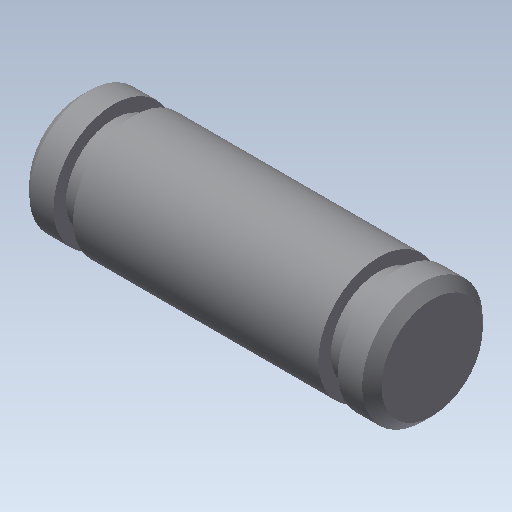
# Autodesk Inventor part: D-12304
Saved by Autodesk Inventor 2020 (Build 240168000, 168)
## iProperties
Created: 2020-01-07
Part Number: D-12304
Material: Generic
Catalog Web Link: www.cadenas.de
Description: Piston Rod Clevis for Original Line Cylinders - Pin-
Vendor: BIMBA
Document SubType Name: Modeling
Designer: psadmin
Manufacturer: BIMBA
Mass: 0.233427 g
Surface Area: 2.57002 cm^2
Volume: 0.233427 cm^3
Density: 1 g/cm^3
Appearance: PSOLRGB-191-191-191
Category: PARTsolutions
Company: BIMBA
PSOL_IDENT_0: {$CADENAS_DATA\23d-libs\bimba\bimba_brand\bimba_imperial\bimba_full_line\original_line_cylinders\acc
PSOL_IDENT_1: essories\piston_rod_clevis_pin.prj},199 {VTYP=3D},{NB=D-12304},{LINA=D-12304},{NN=Piston Rod Clevis
PSOL_IDENT_2: for Original Line Cylinders - Pin},{DATE=23.12.2019 10:36:51},{GEOMDATE=03.04.2013 12:23:00},{VERSIO
PSOL_IDENT_3: N=},{LINEID=20},{WBVAR=},{WBNUMERIC=}  {NB=D-12304},{LINA=D-12304},{KT=DUMMY},{PN=D-12304},{L=0.5460
PSOL_IDENT_4: 0000},{L1=0.38000000},{L2=0.03050000},{L4=0.05250000},{D=0.18700000},{D1=0.14800000},{CH=0.01500000}
PSOL_IDENT_5: ,{R=0.00250000},{COLOR=0.75,0.75,0.75,0.00}
NN: Piston Rod Clevis for Original Line Cylinders - Pin
NB: D-12304
NBSYN: $PN.
LINA: D-12304
PN: D-12304
L: 0.546
L1: 0.38
L2: 0.0305
L4: 0.0525
D: 0.187
D1: 0.148
CH: 0.015
R: 0.0025
SUPPLIER: BIMBA
ARTICLENO: D-12304
BOMINFO: D-12304
CREATOR: CADENAS GmbH
Title: D-12304
Author: Cadenas PARTsolutions
Autodesk Inventor part; units mm, degrees
sketch "Sketch_1" plane through (0, 0, 0) normal (0, 0, 1) x (1, 0, 0)
  line L0 (6.9342, 0) -> (-6.9342, 0)
  line L1 (-6.9342, 0) -> (-6.9342, 1.9939)
  line L2 (-6.9342, 1.9939) -> (-6.5532, 2.3749)
  line L3 (-6.5532, 2.3749) -> (-5.6007, 2.3749)
  line L4 (-5.6007, 2.3749) -> (-5.6007, 1.8796)
  line L5 (-5.6007, 1.8796) -> (-4.826, 1.8796)
  line L6 (-4.826, 1.8796) -> (-4.826, 2.3749)
  line L7 (-4.826, 2.3749) -> (4.826, 2.3749)
  line L8 (4.826, 2.3749) -> (4.826, 1.8796)
  line L9 (4.826, 1.8796) -> (5.6007, 1.8796)
  line L10 (5.6007, 1.8796) -> (5.6007, 2.3749)
  line L11 (5.6007, 2.3749) -> (6.5532, 2.3749)
  line L12 (6.5532, 2.3749) -> (6.9342, 1.9939)
  line L13 (6.9342, 1.9939) -> (6.9342, 0)
  line L14 (6.9342, 0) -> (-6.9342, 0)
  constraints: 30 end point
revolve "Revolution1" add sketch "Sketch_1" angle 360 about axis through (6.9342, 0, 0) along (1, 0, 0)
ref_plane "p1_XY" through (0, 0, 2.3749) normal (1, 0, 0) x (0, 0, -1)
ref_plane "p1_YZ" through (0, 0, 2.3749) normal (0, 0, -1) x (0, 1, 0)
ref_plane "p1_ZX" through (0, 0, 2.3749) normal (0, 1, 0) x (1, 0, 0)
ref_plane "p2_XY" through (0, 0, -2.3749) normal (1, 0, 0) x (0, 0, -1)
ref_plane "p2_YZ" through (0, 0, -2.3749) normal (0, 0, -1) x (0, 1, 0)
ref_plane "p2_ZX" through (0, 0, -2.3749) normal (0, 1, 0) x (1, 0, 0)
ref_plane "pin_XY" through (0, 0, 0) normal (1, 0, 0) x (0, 0, -1)
ref_plane "pin_YZ" through (0, 0, 0) normal (0, 0, -1) x (0, 1, 0)
ref_plane "pin_ZX" through (0, 0, 0) normal (0, 1, 0) x (1, 0, 0)
ref_plane "rr1_XY" through (5.2134, 0, 0) normal (1, 0, 0) x (0, 0, -1)
ref_plane "rr1_YZ" through (5.2134, 0, 0) normal (0, 0, -1) x (0, 1, 0)
ref_plane "rr1_ZX" through (5.2134, 0, 0) normal (0, 1, 0) x (1, 0, 0)
ref_plane "rr2_XY" through (-5.2134, 0, 0) normal (1, 0, 0) x (0, 0, -1)
ref_plane "rr2_YZ" through (-5.2134, 0, 0) normal (0, 0, -1) x (0, 1, 0)
ref_plane "rr2_ZX" through (-5.2134, 0, 0) normal (0, 1, 0) x (1, 0, 0)
ref_plane "w21_XY" through (6.9342, 0, 0) normal (0, 1, 0) x (1, 0, 0)
ref_plane "w21_YZ" through (6.9342, 0, 0) normal (1, 0, 0) x (0, 0, -1)
ref_plane "w21_ZX" through (6.9342, 0, 0) normal (0, 0, -1) x (0, 1, 0)
ref_plane "w22_XY" through (-6.9342, 0, 0) normal (0, 1, 0) x (1, 0, 0)
ref_plane "w22_YZ" through (-6.9342, 0, 0) normal (1, 0, 0) x (0, 0, -1)
ref_plane "w22_ZX" through (-6.9342, 0, 0) normal (0, 0, -1) x (0, 1, 0)
body "Solid1"
